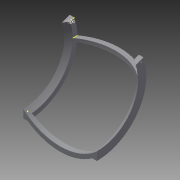
# Autodesk Inventor part: Outer
Saved by Autodesk Inventor 2014 (Build 180170000, 170)
## iProperties
Created: 2014-01-05
Part Number: Outer
Material: Generic
Document SubType Name: Modeling
Designer: Tristan Debrunner
Density: 1 g/cm^3
Appearance: Default
Author: Tristan Debrunner
Autodesk Inventor part; units mm, degrees
ref_plane "YZ Plane" through (0, 0, 0) normal (1, 0, 0) x (0, 1, 0)
ref_plane "XY Plane" through (0, 0, 0) normal (0, 0, 1) x (1, 0, 0)
sketch "Sketch1" plane through (0, 0, 0) normal (0, 0, 1) x (1, 0, 0)
  line L0 (0, 0) -> (0, -45.7841)
  line L1 (25.4, -20.3841) -> (25.4, -45.7841)
  arc A0 (0, 0) -> (25.4, -20.3841) centre (203.2, 227.1845) ccw
  line L2 (25.4, -45.7841) -> (0, -45.7841)
  line L3 (406.4, 0) -> (406.4, -45.7841)
  line L4 (381, -20.3841) -> (381, -45.7841)
  arc A1 (381, -20.3841) -> (406.4, 0) centre (203.2, 227.1845) ccw
  line L5 (381, -45.7841) -> (406.4, -45.7841)
  line L6 (0, 227.1845) -> (560.8643, 227.1845)
  constraints: 14 end point, 4 point on circle, 2 centre point, 2 vertical, 1 perpendicular
revolve "Revolution1" add sketch "Sketch1" angle 110 about axis through (0, 227.1845, 0) along (1, 0, 0)
sketch "Sketch2" plane through (381, -45.7841, 0) normal (0, 0, 1) x (1, 0, 0)
  line L0 (0, 0) -> (0, 25.4) projected
  line L1 (-381, 45.7841) -> (-381, 0) projected
  line L2 (-381, 0) -> (-355.6, 0) projected
  line L3 (-355.6, 0) -> (-355.6, 25.4) projected
  arc A0 (-381, 45.7841) -> (-355.6, 25.4) centre (-177.8, 272.9686) ccw projected
  arc A1 (-355.6, 25.4) -> (0, 25.4) centre (-177.8, 272.9686) ccw
  arc A2 (-355.6, 0) -> (0, 0) centre (-177.8, 247.5686) ccw
  line L4 (0, 0) -> (0, 25.4)
  line L5 (-355.6, 25.4) -> (-355.6, 0)
  line L6 (-381, 350.5841) -> (129.8201, 350.5841)
  dimension "d6" = 304.8
  constraints: 6 end point, 4 point on circle, 2 centre point, 2 collinear, 2 point on line
  measures "d6" radius of A2
revolve "Revolution2" add sketch "Sketch2" angle 4 about axis through (0, 304.8, 0) along (1, 0, 0) contours A2 L3 A1 L0
ref_plane "Work Plane1" through (0, 304.8, 0) normal (0, 1, 0) x (-1, 0, 0)
ref_plane "Work Plane2" through (560.8643, 227.1845, 0) normal (0, 1, 0) x (-1, 0, 0)
sketch "Sketch5" plane through (560.8643, 227.1845, 0) normal (0, 1, 0) x (-1, 0, 0)
  arc A0 (154.4643, -227.1845) -> (179.8643, -247.5686) centre (357.6643, 0) ccw projected
  line L0 (179.8643, -247.5686) -> (179.8643, -272.9686) projected
  line L1 (179.8643, -272.9686) -> (154.4643, -272.9686) projected
  line L2 (154.4643, -272.9686) -> (154.4643, -227.1845) projected
  line L3 (535.4643, -272.9686) -> (535.4643, -247.5686) projected
  arc A1 (535.4643, -247.5686) -> (560.8643, -227.1845) centre (357.6643, 0) ccw projected
  line L4 (560.8643, -227.1845) -> (560.8643, -272.9686) projected
  line L5 (560.8643, -272.9686) -> (535.4643, -272.9686) projected
  arc A2 (179.8643, -247.5686) -> (535.4643, -247.5686) centre (357.6643, 0) ccw
  arc A3 (179.8643, -272.9686) -> (535.4643, -272.9686) centre (357.6643, -25.4) ccw
  line L6 (179.8643, -272.9686) -> (179.8643, -247.5686)
  line L7 (535.4643, -272.9686) -> (535.4643, -247.5686)
  line L8 (357.6643, 0) -> (560.8643, 0)
  dimension "d30" = 304.8
  dimension "d31" = 304.8
  constraints: 6 end point, 4 point on circle, 2 centre point, 2 equal length
  measures "d30" radius of A2
  measures "d31" radius of A3
revolve "Revolution4" add sketch "Sketch5" angle 4 about axis through (203.2, 227.1845, 0) along (-1, 0, 0) contours A2 L3 A3 L0
sketch "Sketch6" plane through (25.4, 227.1845, -247.5686) normal (1, 0, 0) x (0, 0, -1)
  line L0 (0, 0) -> (25.4, 0) projected
  line L1 (-14.9302, 84.6734) -> (8.938, 93.3608) projected
  line L2 (-2.9961, 89.0171) -> (-2.9961, 76.3171)
  point P0 (-247.5686, -227.1845)
  dimension "d33" = 12.7
  constraints: 2 end point, 1 midpoint, 1 perpendicular
  measures "d33" distance of L2.start L2.end
hole "Hole3" at (25.4, 303.5016, -244.5725) direction (1, 0, 0) diameter 6.35 end through all
hole "Hole4" at (25.4, 303.5016, -244.5725) direction (-1, 0, 0) diameter 6.35 end through all
body "Solid1"
